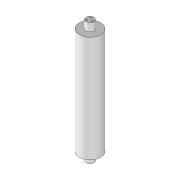
# Autodesk Inventor part: Foerderbandrollen
Saved by Autodesk Inventor 2020 (Build 240168000, 168)
## iProperties
Created: 2020-03-18
Part Number: Foerderbandrollen
Material: Generisch
Document SubType Name: Modeling
Designer: franz
Density: 1 g/cm^3
Appearance: Vorgabe
Author: franz
Autodesk Inventor part; units mm, degrees
ref_plane "YZ Plane" through (0, 0, 0) normal (1, 0, 0) x (0, 1, 0)
ref_plane "XZ Plane" through (0, 0, 0) normal (0, 1, 0) x (-1, 0, 0)
ref_plane "XY Plane" through (0, 0, 0) normal (0, 0, 1) x (1, 0, 0)
sketch "Skizze1" plane through (0, 0, 0) normal (0, 1, 0) x (-1, 0, 0)
  circle A0 centre (0, 0) radius 40
  dimension "d0" = 80
  constraints: 1 centre point, 1 coincident
  measures "d0" diameter of A0
extrude "Extrusion1" add sketch "Skizze1" along normal blind 200
sketch "Skizze2" plane through (0, 0, 0) normal (0, -1, 0) x (1, 0, 0)
  circle A0 centre (0, 0) radius 15
  dimension "d3" = 30
  constraints: 1 centre point, 1 coincident
  measures "d3" diameter of A0
extrude "Extrusion2" add sketch "Skizze2" along normal blind 30
sketch "Skizze3" plane through (0, -30, 0) normal (0, -1, 0) x (1, 0, 0)
  line L0 (0, 0) -> (-7.5, 12.9904)
  circle A0 centre (0, 0) radius 15 projected
  line L1 (0, 0) -> (-7.5, -12.9904)
  line L2 (0, 0) -> (15, 0)
  circle A1 centre (0, 0) radius 10
  point P0 (-5, -8.6603)
  point P1 (-5, 8.6603)
  point P2 (10, 0)
  dimension "d6" = 120
  dimension "d7" = 120
  dimension "d8" = 20
  constraints: 6 end point, 6 point on circle, 3 point on line, 1 centre point, 1 coincident, 1 horizontal
  measures "d6" angle of L2 L1
  measures "d7" angle of L2 L0
  measures "d8" diameter of A1
hole "Bohrung1" at (-5, -30, -8.6603) at (-5, -30, 8.6603) at (10, -30, 0) direction (0, 1, 0) diameter 8 depth 2 tip angle 118
mirror "Spiegeln1" about plane through (0, 200, 0) normal (0, 1, 0) of "Extrusion1", "Extrusion2", "Bohrung1"
